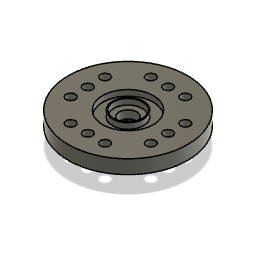
Omnifit_3bar_valve_control_full (Autodesk Fusion 360 archive; units mm, degrees)
design "Servo_round_arm"
Autodesk Fusion 360 part; units mm, degrees
sketch "Sketch1" plane through (0, 0, 0) normal (0, 1, 0) x (1, 0, 0)
  circle A0 centre (0, 0) radius 10.4
  circle A1 centre (0, 0) radius 4.4
  line L0 (7, -7) -> (-7, -7) construction
  line L1 (-7, -7) -> (-7, 7) construction
  line L2 (-7, 7) -> (7, 7) construction
  line L3 (7, 7) -> (7, -7) construction
  line L4 (7, -7) -> (-7, 7) construction
  line L5 (-7, -7) -> (7, 7) construction
  circle A2 centre (0, 0) radius 1.5
  circle A3 centre (0, 0) radius 2.5
  line L6 (0, 10.4) -> (0, -10.4) construction
  circle A4 centre (0, 7) radius 0.8
  circle A5 centre (3, 7) radius 0.8
  circle A6 centre (3, 7) radius 0.8
  circle A7 centre (-3, 7) radius 0.8
  circle A8 centre (-7, 0) radius 0.8
  circle A9 centre (-7, -3) radius 0.8
  circle A10 centre (-7, 3) radius 0.8
  circle A11 centre (0, -7) radius 0.8
  circle A12 centre (3, -7) radius 0.8
  circle A13 centre (-3, -7) radius 0.8
  circle A14 centre (7, 0) radius 0.8
  circle A15 centre (7, 3) radius 0.8
  circle A16 centre (7, -3) radius 0.8
  circle A17 centre (0, 0) radius 2.7
  circle A18 centre (0, 0) radius 4.5
  dimension "d1" = 20.8
  dimension "d2" = 8.8
  dimension "d3" = 14
  dimension "d4" = 3
  dimension "d5" = 5
  dimension "d6" = 1.6
  dimension "d7" = 1.6
  dimension "d8" = 3
  dimension "d9" = 1.6
  dimension "d10" = 1.6
  dimension "d11" = 3
  dimension "d13" = 360
  dimension "d14" = 5.4
  dimension "d15" = 9
  constraint coincident A0.centre A1.centre
  constraint horizontal L0
  constraint perpendicular L0 L1
  constraint parallel L0 L2
  constraint parallel L1 L3
  constraint coincident L4 A0.centre
  constraint coincident L5 A0.centre
  constraint equal L2 L3
  constraint concentric A0 A2
  constraint concentric A2 A3
  constraint coincident A0 L6.start
  constraint coincident A0 L6.end
  constraint vertical L6
  constraint midpoint L2 A4.centre
  constraint coincident L2 A5.centre
  constraint concentric A0 A17
  measures "d1" diameter of A0
  measures "d2" diameter of A1
  measures "d3" distance of L1.end L2.end
  measures "d4" diameter of A2
  measures "d5" diameter of A3
  measures "d6" diameter of A4
  measures "d7" diameter of A5
  measures "d8" distance of A4.centre A5.centre
  measures "d9" diameter of A6
  measures "d10" diameter of A7
  measures "d11" distance of A4.centre A7.centre
  measures "d14" diameter of A17
  measures "d15" diameter of A18
extrude "Extrude1" add sketch "Sketch1" against normal blind 2.4 contours A0 | A1 | A3 | A17 | A18
extrude "Extrude2" add sketch "Sketch1" against normal blind 5.4 contours A1
extrude "Extrude3" cut sketch "Sketch1" against normal blind 1 contours A1 | A3
sketch "Sketch2" plane through (0, -2.4, 0) normal (0, -1, 0) x (1, 0, 0)
  circle A0 centre (0, 0) radius 2.7
  circle A1 centre (0, 0) radius 1.5
sketch "sketch 661" plane through (0, 43, 10.2) normal (0, 1, 0) x (1, 0, 0)
  line L0 (-1.2275, 12.8084, -45.4) -> (-1.1632, 12.9653, -45.4)
  arc A0 through (-0.8109, 12.9664, -45.4) (-1.0223, 12.8955, -45.4) (-1.2275, 12.8084, -45.4)
  line L1 (-0.9631, 13.0412, -45.4) -> (-0.8109, 12.9664, -45.4)
  arc A1 through (-0.9631, 13.0412, -45.4) (-1.0638, 13.005, -45.4) (-1.1632, 12.9653, -45.4)
  line L2 (-1.8161, 12.4389, -45.4) -> (-1.7911, 12.6066, -45.4)
  arc A2 through (-1.4494, 12.692, -45.4) (-1.6376, 12.5725, -45.4) (-1.8161, 12.4389, -45.4)
  line L3 (-1.6151, 12.7281, -45.4) -> (-1.4494, 12.692, -45.4)
  arc A3 through (-1.6151, 12.7281, -45.4) (-1.7042, 12.669, -45.4) (-1.7911, 12.6066, -45.4)
  line L4 (-2.2991, 11.9392, -45.4) -> (-2.315, 12.108, -45.4)
  arc A4 through (-2.0036, 12.2727, -45.4) (-2.1578, 12.1117, -45.4) (-2.2991, 11.9392, -45.4)
  line L5 (-2.1732, 12.2682, -45.4) -> (-2.0036, 12.2727, -45.4)
  arc A5 through (-2.1732, 12.2682, -45.4) (-2.2455, 12.1894, -45.4) (-2.315, 12.108, -45.4)
  line L6 (-2.6485, 11.3384, -45.4) -> (-2.7044, 11.4986, -45.4)
  arc A6 through (-2.4415, 11.733, -45.4) (-2.5526, 11.5397, -45.4) (-2.6485, 11.3384, -45.4)
  line L7 (-2.605, 11.688, -45.4) -> (-2.4415, 11.733, -45.4)
  arc A7 through (-2.605, 11.688, -45.4) (-2.6564, 11.5942, -45.4) (-2.7044, 11.4986, -45.4)
  line L8 (-2.844, 10.6715, -45.4) -> (-2.9366, 10.8136, -45.4)
  arc A8 through (-2.7374, 11.1042, -45.4) (-2.7991, 10.8899, -45.4) (-2.844, 10.6715, -45.4)
  line L9 (-2.8854, 11.0214, -45.4) -> (-2.7374, 11.1042, -45.4)
  arc A9 through (-2.8854, 11.0214, -45.4) (-2.9128, 10.9179, -45.4) (-2.9366, 10.8136, -45.4)
  line L10 (-2.8742, 9.9772, -45.4) -> (-2.9981, 10.093, -45.4)
  arc A10 through (-2.8742, 10.4228, -45.4) (-2.8828, 10.2, -45.4) (-2.8742, 9.9772, -45.4)
  line L11 (-2.9981, 10.307, -45.4) -> (-2.8742, 10.4228, -45.4)
  arc A11 through (-2.9981, 10.307, -45.4) (-3, 10.2, -45.4) (-2.9981, 10.093, -45.4)
  line L12 (-2.7374, 9.2958, -45.4) -> (-2.8854, 9.3786, -45.4)
  arc A12 through (-2.844, 9.7285, -45.4) (-2.7991, 9.5101, -45.4) (-2.7374, 9.2958, -45.4)
  line L13 (-2.9366, 9.5864, -45.4) -> (-2.844, 9.7285, -45.4)
  arc A13 through (-2.9366, 9.5864, -45.4) (-2.9128, 9.4821, -45.4) (-2.8854, 9.3786, -45.4)
  line L14 (-2.4415, 8.667, -45.4) -> (-2.605, 8.712, -45.4)
  arc A14 through (-2.6485, 9.0616, -45.4) (-2.5526, 8.8603, -45.4) (-2.4415, 8.667, -45.4)
  line L15 (-2.7044, 8.9014, -45.4) -> (-2.6485, 9.0616, -45.4)
  arc A15 through (-2.7044, 8.9014, -45.4) (-2.6564, 8.8058, -45.4) (-2.605, 8.712, -45.4)
  line L16 (-2.0036, 8.1273, -45.4) -> (-2.1732, 8.1318, -45.4)
  arc A16 through (-2.2991, 8.4608, -45.4) (-2.1578, 8.2883, -45.4) (-2.0036, 8.1273, -45.4)
  line L17 (-2.315, 8.292, -45.4) -> (-2.2991, 8.4608, -45.4)
  arc A17 through (-2.315, 8.292, -45.4) (-2.2455, 8.2106, -45.4) (-2.1732, 8.1318, -45.4)
  line L18 (-0.5676, 13.0264, -45.4) -> (-0.4676, 13.1633, -45.4)
  arc A18 through (-0.1253, 13.0801, -45.4) (-0.3475, 13.0618, -45.4) (-0.5676, 13.0264, -45.4)
  line L19 (-0.2552, 13.1891, -45.4) -> (-0.1253, 13.0801, -45.4)
  arc A19 through (-0.2552, 13.1891, -45.4) (-0.3616, 13.1781, -45.4) (-0.4676, 13.1633, -45.4)
  line L20 (0.1253, 13.0801, -45.4) -> (0.2552, 13.1891, -45.4)
  arc A20 through (0.5676, 13.0264, -45.4) (0.3475, 13.0618, -45.4) (0.1253, 13.0801, -45.4)
  line L21 (0.4676, 13.1633, -45.4) -> (0.5676, 13.0264, -45.4)
  arc A21 through (0.4676, 13.1633, -45.4) (0.3616, 13.1781, -45.4) (0.2552, 13.1891, -45.4)
  line L22 (0.8109, 12.9664, -45.4) -> (0.9631, 13.0412, -45.4)
  arc A22 through (1.2275, 12.8084, -45.4) (1.0223, 12.8955, -45.4) (0.8109, 12.9664, -45.4)
  line L23 (1.1632, 12.9653, -45.4) -> (1.2275, 12.8084, -45.4)
  arc A23 through (1.1632, 12.9653, -45.4) (1.0638, 13.005, -45.4) (0.9631, 13.0412, -45.4)
  line L24 (1.4494, 12.692, -45.4) -> (1.6151, 12.7281, -45.4)
  arc A24 through (1.8161, 12.4389, -45.4) (1.6376, 12.5725, -45.4) (1.4494, 12.692, -45.4)
  line L25 (1.7911, 12.6066, -45.4) -> (1.8161, 12.4389, -45.4)
  arc A25 through (1.7911, 12.6066, -45.4) (1.7042, 12.669, -45.4) (1.6151, 12.7281, -45.4)
  line L26 (2.0036, 12.2727, -45.4) -> (2.1732, 12.2682, -45.4)
  arc A26 through (2.2991, 11.9392, -45.4) (2.1578, 12.1117, -45.4) (2.0036, 12.2727, -45.4)
  line L27 (2.315, 12.108, -45.4) -> (2.2991, 11.9392, -45.4)
  arc A27 through (2.315, 12.108, -45.4) (2.2455, 12.1894, -45.4) (2.1732, 12.2682, -45.4)
  line L28 (2.4415, 11.733, -45.4) -> (2.605, 11.688, -45.4)
  arc A28 through (2.6485, 11.3384, -45.4) (2.5526, 11.5397, -45.4) (2.4415, 11.733, -45.4)
  line L29 (2.7044, 11.4986, -45.4) -> (2.6485, 11.3384, -45.4)
  arc A29 through (2.7044, 11.4986, -45.4) (2.6564, 11.5942, -45.4) (2.605, 11.688, -45.4)
  line L30 (2.7374, 11.1042, -45.4) -> (2.8854, 11.0214, -45.4)
  arc A30 through (2.844, 10.6715, -45.4) (2.7991, 10.8899, -45.4) (2.7374, 11.1042, -45.4)
  line L31 (2.9366, 10.8136, -45.4) -> (2.844, 10.6715, -45.4)
  arc A31 through (2.9366, 10.8136, -45.4) (2.9128, 10.9179, -45.4) (2.8854, 11.0214, -45.4)
  line L32 (2.8742, 10.4228, -45.4) -> (2.9927, 10.3927, -45.3184)
  arc A32 through (2.8742, 9.9772, -45.4) (2.8828, 10.2, -45.4) (2.8742, 10.4228, -45.4)
  line L33 (2.9981, 10.093, -45.4) -> (2.8742, 9.9772, -45.4)
  arc A33 through (2.9981, 10.093, -45.4) (2.9994, 10.2429, -45.3592) (2.9927, 10.3927, -45.3184)
  line L34 (2.844, 9.7285, -45.4) -> (2.9366, 9.5864, -45.4)
  arc A34 through (2.7374, 9.2958, -45.4) (2.7991, 9.5101, -45.4) (2.844, 9.7285, -45.4)
  line L35 (2.8854, 9.3786, -45.4) -> (2.7374, 9.2958, -45.4)
  arc A35 through (2.8854, 9.3786, -45.4) (2.9128, 9.4821, -45.4) (2.9366, 9.5864, -45.4)
  line L36 (2.6485, 9.0616, -45.4) -> (2.7044, 8.9014, -45.4)
  arc A36 through (2.4415, 8.667, -45.4) (2.5526, 8.8603, -45.4) (2.6485, 9.0616, -45.4)
  line L37 (2.605, 8.712, -45.4) -> (2.4415, 8.667, -45.4)
  arc A37 through (2.605, 8.712, -45.4) (2.6564, 8.8058, -45.4) (2.7044, 8.9014, -45.4)
  line L38 (2.2991, 8.4608, -45.4) -> (2.315, 8.292, -45.4)
  arc A38 through (2.0036, 8.1273, -45.4) (2.1578, 8.2883, -45.4) (2.2991, 8.4608, -45.4)
  line L39 (2.1732, 8.1318, -45.4) -> (2.0036, 8.1273, -45.4)
  arc A39 through (2.1732, 8.1318, -45.4) (2.2455, 8.2106, -45.4) (2.315, 8.292, -45.4)
  line L40 (1.8161, 7.9611, -45.4) -> (1.7911, 7.7934, -45.4)
  arc A40 through (1.4494, 7.708, -45.4) (1.6376, 7.8275, -45.4) (1.8161, 7.9611, -45.4)
  line L41 (1.6151, 7.6719, -45.4) -> (1.4494, 7.708, -45.4)
  arc A41 through (1.6151, 7.6719, -45.4) (1.7042, 7.731, -45.4) (1.7911, 7.7934, -45.4)
  line L42 (1.2275, 7.5916, -45.4) -> (1.1632, 7.4347, -45.4)
  arc A42 through (0.8109, 7.4336, -45.4) (1.0223, 7.5045, -45.4) (1.2275, 7.5916, -45.4)
  line L43 (0.9631, 7.3588, -45.4) -> (0.8109, 7.4336, -45.4)
  arc A43 through (0.9631, 7.3588, -45.4) (1.0638, 7.395, -45.4) (1.1632, 7.4347, -45.4)
  line L44 (0.5676, 7.3736, -45.4) -> (0.4676, 7.2367, -45.4)
  arc A44 through (0.1253, 7.3199, -45.4) (0.3475, 7.3382, -45.4) (0.5676, 7.3736, -45.4)
  line L45 (0.1253, 7.3199, -45.4) -> (0.2552, 7.2109, -45.4)
  arc A45 through (0.2552, 7.2109, -45.4) (0.3616, 7.2219, -45.4) (0.4676, 7.2367, -45.4)
  line L46 (-0.4676, 7.2367, -45.4) -> (-0.5676, 7.3736, -45.4)
  arc A46 through (-0.4676, 7.2367, -45.4) (-0.3616, 7.2219, -45.4) (-0.2552, 7.2109, -45.4)
  line L47 (-0.2552, 7.2109, -45.4) -> (-0.1253, 7.3199, -45.4)
  arc A47 through (-0.5676, 7.3736, -45.4) (-0.3475, 7.3382, -45.4) (-0.1253, 7.3199, -45.4)
  line L48 (-0.8109, 7.4336, -45.4) -> (-0.9631, 7.3588, -45.4)
  arc A48 through (-1.2275, 7.5916, -45.4) (-1.0223, 7.5045, -45.4) (-0.8109, 7.4336, -45.4)
  line L49 (-1.1632, 7.4347, -45.4) -> (-1.2275, 7.5916, -45.4)
  arc A49 through (-1.1632, 7.4347, -45.4) (-1.0638, 7.395, -45.4) (-0.9631, 7.3588, -45.4)
  line L50 (-1.4494, 7.708, -45.4) -> (-1.6151, 7.6719, -45.4)
  arc A50 through (-1.8161, 7.9611, -45.4) (-1.6376, 7.8275, -45.4) (-1.4494, 7.708, -45.4)
  line L51 (-1.7911, 7.7934, -45.4) -> (-1.8161, 7.9611, -45.4)
  arc A51 through (-1.7911, 7.7934, -45.4) (-1.7042, 7.731, -45.4) (-1.6151, 7.6719, -45.4)
  line L52 (-0.5676, 7.3736, -45.4) -> (-0.6641, 7.5056, -45.4)
  arc A52 through (-0.5676, 7.3736, -45.4) (-0.3475, 7.3382, -45.4) (-0.1253, 7.3199, -45.4)
  line L53 (-0.1253, 7.3199, -45.4) -> (0, 7.425, -45.4)
  line L54 (0, 7.425, -45.4) -> (0.1253, 7.3199, -45.4)
  arc A53 through (0.1253, 7.3199, -45.4) (0.3475, 7.3382, -45.4) (0.5676, 7.3736, -45.4)
  line L55 (0.6641, 7.5056, -45.4) -> (0.5676, 7.3736, -45.4)
  line L56 (0.8109, 7.4336, -45.4) -> (0.6641, 7.5056, -45.4)
  arc A54 through (0.8109, 7.4336, -45.4) (1.0223, 7.5045, -45.4) (1.2275, 7.5916, -45.4)
  line L57 (1.2896, 7.7429, -45.4) -> (1.2275, 7.5916, -45.4)
  line L58 (1.4494, 7.708, -45.4) -> (1.2896, 7.7429, -45.4)
  arc A55 through (1.4494, 7.708, -45.4) (1.6376, 7.8275, -45.4) (1.8161, 7.9611, -45.4)
  line L59 (1.8402, 8.1229, -45.4) -> (1.8161, 7.9611, -45.4)
  line L60 (2.0036, 8.1273, -45.4) -> (1.8402, 8.1229, -45.4)
  arc A56 through (2.0036, 8.1273, -45.4) (2.1578, 8.2883, -45.4) (2.2991, 8.4608, -45.4)
  line L61 (2.2838, 8.6236, -45.4) -> (2.2991, 8.4608, -45.4)
  line L62 (2.4415, 8.667, -45.4) -> (2.2838, 8.6236, -45.4)
  arc A57 through (2.4415, 8.667, -45.4) (2.5526, 8.8603, -45.4) (2.6485, 9.0616, -45.4)
  line L63 (2.5947, 9.216, -45.4) -> (2.6485, 9.0616, -45.4)
  line L64 (2.7374, 9.2958, -45.4) -> (2.5947, 9.216, -45.4)
  arc A58 through (2.7374, 9.2958, -45.4) (2.7991, 9.5101, -45.4) (2.844, 9.7285, -45.4)
  line L65 (2.7548, 9.8655, -45.4) -> (2.844, 9.7285, -45.4)
  line L66 (2.8742, 9.9772, -45.4) -> (2.7548, 9.8655, -45.4)
  arc A59 through (2.8742, 9.9772, -45.4) (2.8828, 10.2, -45.4) (2.8742, 10.4228, -45.4)
  line L67 (2.7548, 10.5345, -45.4) -> (2.8742, 10.4228, -45.4)
  line L68 (2.844, 10.6715, -45.4) -> (2.7548, 10.5345, -45.4)
  arc A60 through (2.844, 10.6715, -45.4) (2.7991, 10.8899, -45.4) (2.7374, 11.1042, -45.4)
  line L69 (2.5947, 11.184, -45.4) -> (2.7374, 11.1042, -45.4)
  line L70 (2.6485, 11.3384, -45.4) -> (2.5947, 11.184, -45.4)
  arc A61 through (2.6485, 11.3384, -45.4) (2.5526, 11.5397, -45.4) (2.4415, 11.733, -45.4)
  line L71 (2.2838, 11.7764, -45.4) -> (2.4415, 11.733, -45.4)
  line L72 (2.2991, 11.9392, -45.4) -> (2.2838, 11.7764, -45.4)
  arc A62 through (2.2991, 11.9392, -45.4) (2.1578, 12.1117, -45.4) (2.0036, 12.2727, -45.4)
  line L73 (1.8402, 12.2771, -45.4) -> (2.0036, 12.2727, -45.4)
  line L74 (1.8161, 12.4389, -45.4) -> (1.8402, 12.2771, -45.4)
  arc A63 through (1.8161, 12.4389, -45.4) (1.6376, 12.5725, -45.4) (1.4494, 12.692, -45.4)
  line L75 (1.2896, 12.6571, -45.4) -> (1.4494, 12.692, -45.4)
  line L76 (1.2275, 12.8084, -45.4) -> (1.2896, 12.6571, -45.4)
  arc A64 through (1.2275, 12.8084, -45.4) (1.0223, 12.8955, -45.4) (0.8109, 12.9664, -45.4)
  line L77 (0.6641, 12.8944, -45.4) -> (0.8109, 12.9664, -45.4)
  line L78 (0.5676, 13.0264, -45.4) -> (0.6641, 12.8944, -45.4)
  arc A65 through (0.5676, 13.0264, -45.4) (0.3475, 13.0618, -45.4) (0.1253, 13.0801, -45.4)
  line L79 (0, 12.975, -45.4) -> (0.1253, 13.0801, -45.4)
  line L80 (-0.1253, 13.0801, -45.4) -> (0, 12.975, -45.4)
  arc A66 through (-0.1253, 13.0801, -45.4) (-0.3475, 13.0618, -45.4) (-0.5676, 13.0264, -45.4)
  line L81 (-0.6641, 12.8944, -45.4) -> (-0.5676, 13.0264, -45.4)
  line L82 (-0.8109, 12.9664, -45.4) -> (-0.6641, 12.8944, -45.4)
  arc A67 through (-0.8109, 12.9664, -45.4) (-1.0223, 12.8955, -45.4) (-1.2275, 12.8084, -45.4)
  line L83 (-1.2896, 12.6571, -45.4) -> (-1.2275, 12.8084, -45.4)
  line L84 (-1.4494, 12.692, -45.4) -> (-1.2896, 12.6571, -45.4)
  arc A68 through (-1.4494, 12.692, -45.4) (-1.6376, 12.5725, -45.4) (-1.8161, 12.4389, -45.4)
  line L85 (-1.8402, 12.2771, -45.4) -> (-1.8161, 12.4389, -45.4)
  line L86 (-2.0036, 12.2727, -45.4) -> (-1.8402, 12.2771, -45.4)
  arc A69 through (-2.0036, 12.2727, -45.4) (-2.1578, 12.1117, -45.4) (-2.2991, 11.9392, -45.4)
  line L87 (-2.2838, 11.7764, -45.4) -> (-2.2991, 11.9392, -45.4)
  line L88 (-2.4415, 11.733, -45.4) -> (-2.2838, 11.7764, -45.4)
  arc A70 through (-2.4415, 11.733, -45.4) (-2.5526, 11.5397, -45.4) (-2.6485, 11.3384, -45.4)
  line L89 (-2.5947, 11.184, -45.4) -> (-2.6485, 11.3384, -45.4)
  line L90 (-2.7374, 11.1042, -45.4) -> (-2.5947, 11.184, -45.4)
  arc A71 through (-2.7374, 11.1042, -45.4) (-2.7991, 10.8899, -45.4) (-2.844, 10.6715, -45.4)
  line L91 (-2.7548, 10.5345, -45.4) -> (-2.844, 10.6715, -45.4)
  line L92 (-2.8742, 10.4228, -45.4) -> (-2.7548, 10.5345, -45.4)
  arc A72 through (-2.8742, 10.4228, -45.4) (-2.8828, 10.2, -45.4) (-2.8742, 9.9772, -45.4)
  line L93 (-2.7548, 9.8655, -45.4) -> (-2.8742, 9.9772, -45.4)
  line L94 (-2.844, 9.7285, -45.4) -> (-2.7548, 9.8655, -45.4)
  arc A73 through (-2.844, 9.7285, -45.4) (-2.7991, 9.5101, -45.4) (-2.7374, 9.2958, -45.4)
  line L95 (-2.5947, 9.216, -45.4) -> (-2.7374, 9.2958, -45.4)
  line L96 (-2.6485, 9.0616, -45.4) -> (-2.5947, 9.216, -45.4)
  arc A74 through (-2.6485, 9.0616, -45.4) (-2.5526, 8.8603, -45.4) (-2.4415, 8.667, -45.4)
  line L97 (-2.2838, 8.6236, -45.4) -> (-2.4415, 8.667, -45.4)
  line L98 (-2.2991, 8.4608, -45.4) -> (-2.2838, 8.6236, -45.4)
  arc A75 through (-2.2991, 8.4608, -45.4) (-2.1578, 8.2883, -45.4) (-2.0036, 8.1273, -45.4)
  line L99 (-1.8402, 8.1229, -45.4) -> (-2.0036, 8.1273, -45.4)
  line L100 (-1.8161, 7.9611, -45.4) -> (-1.8402, 8.1229, -45.4)
  arc A76 through (-1.8161, 7.9611, -45.4) (-1.6376, 7.8275, -45.4) (-1.4494, 7.708, -45.4)
  line L101 (-1.2896, 7.7429, -45.4) -> (-1.4494, 7.708, -45.4)
  line L102 (-1.2275, 7.5916, -45.4) -> (-1.2896, 7.7429, -45.4)
  arc A77 through (-1.2275, 7.5916, -45.4) (-1.0223, 7.5045, -45.4) (-0.8109, 7.4336, -45.4)
  line L103 (-0.6641, 7.5056, -45.4) -> (-0.8109, 7.4336, -45.4)
  circle A78 through (2.7, 10.2, -45.4) (-1.35, 12.5383, -45.4) (-1.35, 7.8617, -45.4)
  circle A79 through (2.7, 10.2, -45.4) (-1.35, 12.5383, -45.4) (-1.35, 7.8617, -45.4)
  spline S0 degree 3 poles (0.9444, 9.2556, -45.4) (0.8293, 9.1227, -45.4) (0.6891, 9.0138, -45.4) (0.3708, 8.8528, -45.4) (0.195, 8.804, -45.4) (-0.1702, 8.7752, -45.4) (-0.3563, 8.7973, -45.4) (-0.7145, 8.9122, -45.4) (-0.8826, 9.0057, -45.4) (-1.1277, 9.2122, -45.4) (-1.2156, 9.3085, -45.4) (-1.3657, 9.5231, -45.4) (-1.4269, 9.6408, -45.4) (-1.4722, 9.7648, -45.4) knots 0 0 0 0 0.05274982 0.05274982 0.10693187 0.10693187 0.16254549 0.16254549 0.21959006 0.21959006 0.25846244 0.25846244 0.29797509 0.29797509 0.29797509 0.29797509
  arc A80 through (-0.7333, 11.5487, -45.4) (-1.4183, 10.7875, -45.4) (-1.4722, 9.7648, -45.4)
  spline S1 degree 3 poles (-0.7333, 11.5487, -45.4) (-0.5545, 11.6318, -45.4) (-0.3614, 11.6796, -45.4) (0.0275, 11.6975, -45.4) (0.2195, 11.6691, -45.4) (0.5768, 11.5412, -45.4) (0.7394, 11.4446, -45.4) (1.0141, 11.1972, -45.4) (1.1249, 11.05, -45.4) (1.2555, 10.7784, -45.4) (1.293, 10.6651, -45.4) (1.337, 10.4335, -45.4) (1.344, 10.3165, -45.4) (1.3355, 10.2, -45.4) knots 0 0 0 0 0.05914457 0.05914457 0.11685508 0.11685508 0.17313094 0.17313094 0.22797152 0.22797152 0.26373039 0.26373039 0.29884833 0.29884833 0.29884833 0.29884833
  arc A81 through (0.9444, 9.2556, -45.4) (1.2339, 9.6889, -45.4) (1.3356, 10.2, -45.4)
extrude "Extrude4" cut sketch "sketch 661" against normal blind 3 contours L0 A0 L1 A1 A67 | A0 A2 A4 A6 A8 A10 A12 A14 A16 A18 A20 A22 A24 A26 A28 A30 A32 A34 A36 A38 A40 A42 A44 A47 A48 A50 L52 A52 L53 L54 A53 L55 L56 A54 L57 L58 A55 L59 L60 A56 L61 L62 A57 L63 L64 A58 L65 L66 A59 L67 L68 A60 L69 L70 A61 L71 L72 A62 L73 L74 A63 L75 L76 A64 L77 L78 A65 L79 L80 A66 L81 L82 A67 L83 L84 A68 L85 L86 A69 L87 L88 A70 L89 L90 A71 L91 L92 A72 L93 L94 A73 L95 L96 A74 L97 L98 A75 L99 L100 A76 L101 L102 A77 L103 | L2 A2 L3 A3 A68 | L18 A18 L19 A19 A66 | L4 A4 L5 A5 A69 | L20 A20 L21 A21 A65 | L6 A6 L7 A7 A70 | L22 A22 L23 A23 A64 | L8 A8 L9 A9 A71 | L24 A24 L25 A25 A63 | L10 A10 L11 A11 A72 | L26 A26 L27 A27 A62 | L12 A12 L13 A13 A73 | L28 A28 L29 A29 A61 | L14 A14 L15 A15 A74 | L30 A30 L31 A31 A60 | L16 A16 L17 A17 A75 | L50 A50 L51 A51 A76 | L34 A34 L35 A35 A58 | L48 A48 L49 A49 A77 | L36 A36 L37 A37 A57 | L46 A46 L47 A47 A52 | L38 A38 L39 A39 A56 | L44 A44 L45 A45 A53 | L40 A40 L41 A41 A55 | L42 A42 L43 A43 A54 in plane through (0, -2.4, 10.2) normal (0, 1, 0)
